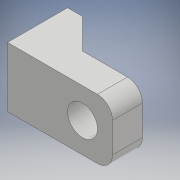
# Autodesk Inventor part: 2
Saved by Autodesk Inventor 2017 (Build 210142000, 142)
## iProperties
Part Number: 2
Material: 一般
Document SubType Name: Modeling
Designer: Brian
Density: 1 g/cm^3
Appearance: 預設
Author: Brian
Autodesk Inventor part; units mm, degrees
ref_plane "YZ Plane" through (0, 0, 0) normal (1, 0, 0) x (0, 1, 0)
ref_plane "XZ Plane" through (0, 0, 0) normal (0, 1, 0) x (-1, 0, 0)
ref_plane "XY Plane" through (0, 0, 0) normal (0, 0, 1) x (1, 0, 0)
sketch "草圖1" plane through (0, 0, 0) normal (0, 1, 0) x (-1, 0, 0)
  line L0 (0, 0) -> (-70, 0)
  line L1 (-70, 0) -> (-70, -40)
  line L2 (-70, -40) -> (0, -40)
  line L3 (0, -40) -> (0, 0)
  dimension "d0" = 40
  dimension "d1" = 70
  constraints: 8 end point, 2 parallel, 1 horizontal, 1 perpendicular
  measures "d0" distance of L2.end L0.start
  measures "d1" distance of L1.end L2.end
extrude "擠出1" add sketch "草圖1" along normal blind 20
sketch "草圖2" plane through (0, 0, 0) normal (0, 0, 1) x (1, 0, 0)
  line L0 (0, 20) -> (70, 20) projected
  line L1 (0, 20) -> (10, 20)
  line L2 (10, 20) -> (10, 40)
  line L3 (10, 40) -> (0, 40)
  line L4 (0, 40) -> (0, 20)
  point P0 (0, 0)
  dimension "d4" = 10
  dimension "d5" = 20
  constraints: 8 end point, 2 parallel, 1 horizontal, 1 perpendicular
  measures "d4" distance of L2.end L3.end
  measures "d5" distance of L3.end L0.start
extrude "擠出2" add sketch "草圖2" against normal up to surface (40 mm away)
sketch "草圖3" plane through (70, 0, -40) normal (0, 0, -1) x (-1, 0, 0)
  line L0 (60, 20) -> (60, 40) projected
  line L1 (60, 20) -> (40, 20)
  line L2 (40, 20) -> (40, 40)
  line L3 (40, 40) -> (60, 40)
  line L4 (60, 40) -> (60, 20)
  point P0 (70, 0)
  dimension "d8" = 20
  dimension "d9" = 20
  constraints: 8 end point, 2 parallel, 1 horizontal, 1 perpendicular
  measures "d8" distance of L2.end L3.end
  measures "d9" distance of L1.end L2.end
extrude "擠出3" add sketch "草圖3" against normal blind 10
sketch "草圖4" plane through (0, 0, 0) normal (0, 0, 1) x (1, 0, 0)
  line L0 (30, 20) -> (10, 20) projected
  line L1 (30, 20) -> (30, 40) projected
  line L2 (30, 40) -> (10, 40) projected
  line L3 (10, 20) -> (10, 40) projected
  point P0 (0, 0)
extrude "擠出4" add sketch "草圖4" against normal blind 10
chamfer "倒角1" distance 20 angle 45 1 edges at (30, 40, -5)
fillet "圓角1" radius 10 2 edges at (70, 10, 0) (70, 10, -40)
sketch "草圖5" plane through (0, 20, 0) normal (0, 1, 0) x (1, 0, 0)
  circle A0 centre (50, 20) radius 10
  line L0 (30, 0) -> (60, 0) projected
  line L1 (70, 10) -> (70, 30) projected
  point P0 (0, 0)
  dimension "d18" = 20
  dimension "d19" = 20
  dimension "d20" = 20
  constraints: 1 centre point
  measures "d18" distance from line of L0 A0.centre
  measures "d19" diameter of A0
  measures "d20" distance from line of L1 A0.centre
extrude "擠出5" cut sketch "草圖5" against normal through all
